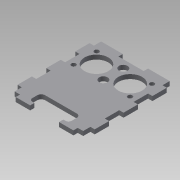
# Autodesk Inventor part: srf depan
Saved by Autodesk Inventor 2015 SP1 (Build 190203100, 203)
## iProperties
Created: 2015-02-14
Part Number: srf depan
Material: Generic
Document SubType Name: Modeling
Designer: Rafi Kurnia Putra
Density: 1 g/cm^3
Appearance: Default
Author: Rafi Kurnia Putra
Autodesk Inventor part; units mm, degrees
ref_plane "YZ Plane" through (0, 0, 0) normal (1, 0, 0) x (0, 1, 0)
ref_plane "XZ Plane" through (0, 0, 0) normal (0, 1, 0) x (-1, 0, 0)
ref_plane "XY Plane" through (0, 0, 0) normal (0, 0, 1) x (1, 0, 0)
sketch "Sketch1" plane through (0, 0, 0) normal (0, 0, 1) x (1, 0, 0)
  line L0 (23.778, 63) -> (8.7494, 62.999)
  line L1 (8.7496, 59.9961) -> (8.7494, 62.999)
  line L2 (-8.7499, 59.9964) -> (8.7496, 59.9961)
  line L3 (-8.7498, 62.9964) -> (-8.7499, 59.9964)
  line L4 (-8.7498, 62.9964) -> (-23.7781, 62.9967)
  circle A0 centre (11.7, 47.6838) radius 8.25
  circle A1 centre (-11.7, 47.6838) radius 8.25
  circle A2 centre (0.0002, 40.7838) radius 2.95
  circle A3 centre (19.375, 39.8838) radius 1.5875
  circle A4 centre (-19.375, 55.4838) radius 1.5875
  line L5 (10.98, 11.2972) -> (-10.98, 11.2972)
  arc A5 (13.638, 8.6392) -> (10.98, 11.2972) centre (10.98, 8.6392) ccw
  arc A6 (-10.98, 11.2972) -> (-13.638, 8.6392) centre (-10.98, 8.6392) ccw
  line L6 (-0.0001, 27) -> (-7.6501, 27) construction
  line L7 (-7.6501, 27) -> (-0.0001, 27) construction
  line L8 (-0.0001, 34) -> (-0.0001, 27) construction
  line L9 (10, 0) -> (20, 0)
  line L10 (-20, 0) -> (-10, 0)
  line L11 (-5, 0) -> (5, 0) construction
  line L12 (20, 0) -> (20, 3.0003)
  line L13 (20, 3.0003) -> (23.778, 3)
  line L14 (10, 0) -> (10, 3.0012)
  line L15 (-10, 3.0012) -> (-10, 0)
  line L16 (-20, 0) -> (-20, 3)
  line L17 (-20, 3) -> (-23.7781, 3)
  line L18 (13.638, 8.6392) -> (13.638, 5.0012)
  line L19 (-13.638, 8.6392) -> (-13.638, 5.0012)
  line L20 (11.638, 3.0012) -> (10, 3.0012)
  line L21 (-10, 3.0012) -> (-11.638, 3.0012)
  arc A7 (11.638, 3.0012) -> (13.638, 5.0012) centre (11.638, 5.0012) ccw
  arc A8 (-13.638, 5.0012) -> (-11.638, 3.0012) centre (-11.638, 5.0012) ccw
  line L22 (23.778, 28) -> (26.778, 28)
  line L23 (26.778, 28) -> (26.778, 38)
  line L24 (26.778, 38) -> (23.778, 38)
  line L25 (23.778, 48) -> (26.778, 48)
  line L26 (26.778, 48) -> (26.778, 58)
  line L27 (26.778, 58) -> (23.778, 58)
  line L28 (23.778, 8) -> (26.778, 8)
  line L29 (26.778, 8) -> (26.778, 18)
  line L30 (26.778, 18) -> (23.778, 18)
  line L31 (23.778, 28) -> (26.778, 28)
  line L32 (26.778, 28) -> (26.778, 38)
  line L33 (26.778, 38) -> (23.778, 38)
  line L34 (23.778, 48) -> (23.778, 38)
  line L35 (23.778, 28) -> (23.778, 18)
  line L36 (23.778, 8) -> (23.778, 3)
  line L37 (-23.7781, 28) -> (-26.7781, 28)
  line L38 (-26.7781, 28) -> (-26.7781, 38)
  line L39 (-26.7781, 38) -> (-23.7781, 38)
  line L40 (-26.7781, 48) -> (-26.7781, 58)
  line L41 (-26.7781, 58) -> (-23.7781, 58)
  line L42 (-23.7781, 48) -> (-26.7781, 48)
  line L43 (-26.7781, 8) -> (-26.7781, 18)
  line L44 (-26.7781, 18) -> (-23.7781, 18)
  line L45 (-23.7781, 8) -> (-26.7781, 8)
  line L46 (-26.7781, 28) -> (-26.7781, 38)
  line L47 (-26.7781, 38) -> (-23.7781, 38)
  line L48 (-23.7781, 28) -> (-26.7781, 28)
  line L49 (-23.7781, 48) -> (-23.7781, 38)
  line L50 (-23.7781, 28) -> (-23.7781, 18)
  circle A9 centre (0.0002, 54.5838) radius 2.95
  line L51 (0.0002, 50) -> (0.0002, 45) construction
  line L52 (10, 47.5) -> (6, 47.5) construction
  circle A10 centre (19.375, 55.1162) radius 1.5875
  circle A11 centre (-19.375, 39.5162) radius 1.5875
  line L53 (-23.7781, 3) -> (-23.7781, 8)
  line L54 (23.778, 63) -> (23.778, 58)
  line L55 (-23.7781, 62.9967) -> (-23.7781, 58)
  point P0 (0, 0)
  point P1 (0, 1.5)
  point P2 (15, 0)
  point P3 (15, 1.5)
  point P4 (-15, 0)
  point P5 (-15, 1.5)
  point P6 (0, 0)
  point P7 (0, 1.5)
  point P8 (13.638, 3.0012)
  dimension "d4" = 15
  dimension "d7" = 15
  dimension "d11" = 2
  dimension "d12" = 3
  dimension "d16" = 20
  dimension "d19" = 20
  dimension "d46" = 7.675
  dimension "d47" = 7.675
  constraints: 112 end point, 18 symmetric about line, 12 centre point, 8 point on circle, 8 vertical, 7 horizontal, 4 tangent, 3 collinear, 3 parallel, 3 point on line, 2 perpendicular, 1 equal radius, 38 other
  measures "d4" distance of point (0, 0) point (15, 0)
  measures "d7" distance of point (0, 0) point (-15, 0)
  measures "d11" radius of A7
  measures "d12" distance of L24.end L23.end
  measures "d16" distance of L22.end L26.start
  measures "d19" distance of L22.end L29.start
  measures "d46" horizontal distance of A4.centre A1.centre
  measures "d47" horizontal distance of A0.centre A3.centre
extrude "Extrusion1" add sketch "Sketch1" along normal blind 3
body "Solid1"
